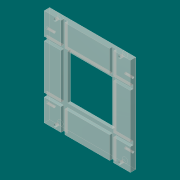
# Autodesk Inventor part: back
Saved by Autodesk Inventor 2016 (Build 200138000, 138)
## iProperties
Created: 2015-10-13
Part Number: back
Material: PC/ABS Plastic
Document SubType Name: Modeling
Designer: Sawaiz
Density: 0.357273 g/cm^3
Appearance: Clear
Author: Sawaiz
Autodesk Inventor part; units mm, degrees
ref_plane "YZ Plane" through (0, 0, 0) normal (1, 0, 0) x (0, 1, 0)
ref_plane "XZ Plane" through (0, 0, 0) normal (0, 1, 0) x (-1, 0, 0)
ref_plane "XY Plane" through (0, 0, 0) normal (0, 0, 1) x (1, 0, 0)
sketch "Sketch1" plane through (0, 0, 0) normal (1, 0, 0) x (0, 1, 0)
  line L0 (-50, -56.35) -> (50, -56.35)
  line L1 (50, -56.35) -> (50, 56.35)
  line L2 (50, 56.35) -> (-50, 56.35)
  line L3 (-50, 56.35) -> (-50, -56.35)
  line L4 (-50, -56.35) -> (50, 56.35) construction
  line L5 (50, -56.35) -> (-50, 56.35) construction
  point P0 (0, 0)
  dimension "d0" = 100
  dimension "d1" = 112.7
  constraints: 12 end point, 2 midpoint, 2 parallel, 1 horizontal, 1 perpendicular
  measures "d0" distance of L2.end L1.end
  measures "d1" distance of L1.end L0.end
extrude "Extrusion1" add sketch "Sketch1" along normal blind 6.35
sketch "Sketch2" plane through (6.35, 0, 0) normal (1, 0, 0) x (0, 0, -1)
  line L0 (-26, 26) -> (26, 26)
  line L1 (26, 26) -> (26, -26)
  line L2 (26, -26) -> (-26, -26)
  line L3 (-26, -26) -> (-26, 26)
  line L4 (-26, 26) -> (26, -26) construction
  line L5 (26, 26) -> (-26, -26) construction
  point P0 (0, 0)
  dimension "d4" = 52
  dimension "d5" = 52
  constraints: 12 end point, 2 midpoint, 2 parallel, 1 horizontal, 1 perpendicular
  measures "d4" distance of L1.end L2.end
  measures "d5" distance of L0.end L1.end
extrude "Extrusion2" cut sketch "Sketch2" against normal through all
sketch "Sketch3" plane through (6.35, 0, 0) normal (1, 0, 0) x (0, 0, -1)
  line L0 (-26, -26) -> (-26, 26) projected
  line L1 (-26, 26) -> (26, 26) projected
  line L2 (26, 26) -> (26, -26) projected
  line L3 (26, -26) -> (-26, -26) projected
  line L4 (56.35, -50) -> (56.35, 50) projected
  line L5 (56.35, 50) -> (-56.35, 50) projected
  line L6 (-56.35, 50) -> (-56.35, -50) projected
  line L7 (-56.35, -50) -> (56.35, -50) projected
  line L8 (-56.35, 30.5) -> (56.35, 30.5)
  line L9 (56.35, 30.5) -> (56.35, 26)
  line L10 (56.35, 26) -> (-56.35, 26)
  line L11 (-56.35, 26) -> (-56.35, 30.5)
  line L12 (-56.35, 30.5) -> (56.35, 26) construction
  line L13 (56.35, 30.5) -> (-56.35, 26) construction
  line L14 (-56.35, -30.5) -> (56.35, -30.5)
  line L15 (56.35, -30.5) -> (56.35, -26)
  line L16 (56.35, -26) -> (-56.35, -26)
  line L17 (-56.35, -26) -> (-56.35, -30.5)
  line L18 (-56.35, -30.5) -> (56.35, -26) construction
  line L19 (56.35, -30.5) -> (-56.35, -26) construction
  line L20 (56.35, 50) -> (-56.35, 50) projected
  line L21 (-30.5, 50) -> (-26, 50)
  line L22 (-26, 50) -> (-26, -50)
  line L23 (-26, -50) -> (-30.5, -50)
  line L24 (-30.5, -50) -> (-30.5, 50)
  line L25 (-56.35, -50) -> (56.35, -50) projected
  line L26 (26, -50) -> (30.5, -50)
  line L27 (30.5, -50) -> (30.5, 50)
  line L28 (30.5, 50) -> (26, 50)
  line L29 (26, 50) -> (26, -50)
  point P0 (0, 28.25)
  point P1 (0, -28.25)
  dimension "d12" = 4.5
  dimension "d13" = 4.5
  dimension "d14" = 4.5
  dimension "d15" = 4.5
  constraints: 40 end point, 8 parallel, 6 collinear, 6 point on line, 4 horizontal, 4 midpoint, 4 perpendicular
  measures "d12" distance between parallel lines of L14 L16
  measures "d13" distance between parallel lines of L8 L10
  measures "d14" distance between parallel lines of L22 L24
  measures "d15" distance between parallel lines of L27 L29
extrude "Extrusion3" cut sketch "Sketch3" against normal blind 3.175 contours L16 L24 L10 L0 | L22 L14 L24 L16 | L3 L29 L14 L22 | L22 L8 L29 L1 | L10 L24 L8 L22 | L2 L10 L27 L16 | L16 L27 L14 L29 | L24 L14 L6 L16 | L22 L7 L24 L14 | L29 L8 L27 L10 | L10 L6 L8 L24 | L8 L24 L5 L22 | L16 L4 L14 L27 | L14 L27 L7 L29 | L27 L8 L4 L10 | L29 L5 L27 L8
sketch "Sketch4" plane through (0, 0, 0) normal (-1, 0, 0) x (0, 0, 1)
  line L0 (26, 26) -> (26, -26) projected
  line L1 (26, -26) -> (-26, -26) projected
  line L2 (-26, -26) -> (-26, 26) projected
  line L3 (-26, 26) -> (26, 26) projected
  line L4 (-56.35, -50) -> (-56.35, 50) projected
  line L5 (56.35, -50) -> (-56.35, -50) projected
  line L6 (56.35, 50) -> (56.35, -50) projected
  line L7 (-56.35, 50) -> (56.35, 50) projected
  line L8 (53.175, 50) -> (53.175, -50)
  line L9 (56.35, 50) -> (56.35, -50) projected
  line L10 (-53.175, 50) -> (-53.175, -50)
  line L11 (-56.35, 50) -> (56.35, 50) projected
  point P0 (0, 0)
  point P1 (-53.175, 37.5)
  point P2 (-53.175, 12.5)
  point P3 (-53.175, -12.5)
  point P4 (-53.175, -37.5)
  point P5 (53.175, -37.5)
  point P6 (53.175, -12.5)
  point P7 (53.175, 12.5)
  point P8 (53.175, 37.5)
  dimension "d16" = 3.175
  dimension "d18" = 3.175
  dimension "d20" = 12.5
  dimension "d21" = 25
  dimension "d22" = 25
  dimension "d23" = 25
  dimension "d33" = 12.5
  dimension "d34" = 12.5
  dimension "d35" = 25
  dimension "d36" = 25
  constraints: 12 point on line, 4 end point, 2 parallel, 1 perpendicular
  measures "d16" distance between parallel lines of L6 L8
  measures "d18" distance between parallel lines of L4 L10
  measures "d20" distance from line of L7 point (53.175, 37.5)
  measures "d21" distance of point (53.175, 12.5) point (53.175, 37.5)
  measures "d22" distance of point (53.175, -12.5) point (53.175, 12.5)
  measures "d23" distance of point (53.175, -12.5) point (53.175, -37.5)
  measures "d33" vertical distance of point (0, 0) point (-53.175, -12.5)
  measures "d34" vertical distance of point (0, 0) point (-53.175, 12.5)
  measures "d35" distance of point (-53.175, 12.5) point (-53.175, 37.5)
  measures "d36" distance of point (-53.175, -12.5) point (-53.175, -37.5)
hole "Hole1" at (0, 37.5, -53.175) at (0, -37.5, -53.175) at (0, -37.5, 53.175) at (0, 37.5, 53.175) direction (1, 0, 0) diameter 3.2 end through all countersink diameter 6.3 countersink angle 90 clearance for "Flat Head Machine Screw" size "M3" standard "Ansi Metric M Profile"
sketch "Sketch5" plane through (0, 50, 56.35) normal (0, 1, 0) x (1, 0, 0)
  line L0 (3.175, 86.85) -> (6.35, 86.85) projected
  line L1 (6.35, 112.7) -> (6.35, 86.85) projected
  line L2 (0, 112.7) -> (6.35, 112.7) projected
  line L3 (0, 112.7) -> (0, 0) projected
  line L4 (0, 0) -> (6.35, 0) projected
  line L5 (6.35, 25.85) -> (6.35, 0) projected
  line L6 (6.35, 25.85) -> (3.175, 25.85) projected
  line L7 (3.175, 25.85) -> (3.175, 30.35) projected
  line L8 (3.175, 30.35) -> (6.35, 30.35) projected
  line L9 (6.35, 82.35) -> (6.35, 30.35) projected
  line L10 (6.35, 82.35) -> (3.175, 82.35) projected
  line L11 (3.175, 82.35) -> (3.175, 86.85) projected
  line L12 (0, 0) -> (6.35, 0) projected
  line L13 (3.175, 0) -> (3.175, 112.7)
  point P0 (0, 56.35)
  point P1 (3.175, 18.85)
  point P2 (3.175, 43.85)
  point P3 (3.175, 68.85)
  point P4 (3.175, 93.85)
  dimension "d48" = 3.175
  dimension "d49" = 12.5
  dimension "d50" = 12.5
  dimension "d51" = 25
  dimension "d52" = 25
  constraints: 4 point on line, 2 end point, 2 midpoint, 1 vertical
  measures "d48" distance between parallel lines of L3 L13
  measures "d49" vertical distance of point (0, 56.35) point (3.175, 68.85)
  measures "d50" vertical distance of point (0, 56.35) point (3.175, 43.85)
  measures "d51" distance of point (3.175, 43.85) point (3.175, 18.85)
  measures "d52" distance of point (3.175, 93.85) point (3.175, 68.85)
hole "Hole2" at (3.175, 50, 37.5) at (3.175, 50, -37.5) direction (0, -1, 0) diameter 2.459 depth 8.8 tip angle 118 thread size "M3x0.5" class "6H" standard "ANSI Metric M Profile"
mirror "Mirror1" about plane through (0, 0, 0) normal (0, 1, 0) of "Hole2"
equation "\"d0\" = width"
equation "\"d1\" = height + 2 * acrylicThickness"
equation "\"d2\" = acrylicThickness"
equation "\"d4\" = detectorHeight"
equation "\"d5\" = detectorWidth"
equation "\"d12\" = 1.5 * mirrorThickness"
equation "\"d13\" = 1.5 * mirrorThickness"
equation "\"d14\" = 1.5 * mirrorThickness"
equation "\"d15\" = 1.5 * mirrorThickness"
equation "\"d10\" = 0.5 * acrylicThickness"
equation "\"d16\" = 0.5 * acrylicThickness"
equation "\"d18\" = 0.5 * acrylicThickness"
equation "\"d20\" = 0.125 * width"
equation "\"d21\" = 0.25 * width"
equation "\"d22\" = 0.25 * width"
equation "\"d23\" = 0.25 * width"
equation "\"d33\" = 0.125 * width"
equation "\"d34\" = 0.125 * width"
equation "\"d35\" = 0.25 * width"
equation "\"d36\" = 0.25 * width"
equation "\"d48\" = 0.5 * acrylicThickness"
equation "\"d49\" = 0.125 * height"
equation "\"d50\" = 0.125 * height"
equation "\"d51\" = 0.25 * height"
equation "\"d52\" = 0.25 * height"
equation "\"acrylicThickness\" = 6.35"
equation "\"width\" = 100"
equation "\"mirrorAngle\" = 17deg"
equation "\"detectorWidth\" = 52"
equation "\"detectorHeight\" = 52"
equation "\"mirrorThickness\" = 3"
equation "\"fresnelThickness\" = 0.1"
equation "\"ior\" = 1.49"
equation "\"focalLength\" = 76.2"
equation "\"fresnelAngle\" = 90deg"
equation "\"centerThickness\" = 1.524"
equation "\"fresnelEffectiveDiameter\" = 76.2"
equation "\"height\" = 100"
body "Solid1"
